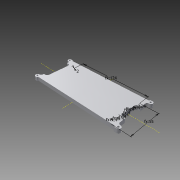
# Autodesk Inventor part: Heatsink
Saved by Autodesk Inventor 2016 (Build 200138000, 138)
## iProperties
Created: 2015-06-09
Part Number: Heatsink
Material: Aluminum 6061
Document SubType Name: Modeling
Designer: Yann
Density: 2.7 g/cm^3
Appearance: Aluminum - Flat
Mass: 133.784 g
Surface Area: 224.248 cm^2
Volume: 49.5496 cm^3
Author: Yann
Autodesk Inventor part; units mm, degrees
ref_plane "YZ Plane" through (0, 0, 0) normal (1, 0, 0) x (0, 1, 0)
ref_plane "XZ Plane" through (0, 0, 0) normal (0, 1, 0) x (-1, 0, 0)
ref_plane "XY Plane" through (0, 0, 0) normal (0, 0, 1) x (1, 0, 0)
sketch "Sketch1" plane through (0, 0, 0) normal (0, 0, 1) x (1, 0, 0)
  line L0 (0, 160210.1999) -> (0, -160210.1999) construction
  line L1 (-160320.9849, 0) -> (160320.9849, 0) construction
  line L2 (0, -32.5) -> (-72, -32.5)
  line L3 (-72, -32.5) -> (-72, -34.5)
  circle A0 centre (-75.5, -31) radius 1.5
  line L4 (-72, -34.5) -> (-75.5, -34.5)
  arc A1 (-75.7128, -27.5065) -> (-75.5, -34.5) centre (-75.5, -31) ccw
  line L5 (-72, -24.3936) -> (-72, 0) construction
  line L6 (-75.7128, -27.5065) -> (-72, -27.2803) construction
  line L7 (-72, -27.2803) -> (-72, -24.3936) construction
  spline S0 degree 2 poles (-75.7128, -27.5065) (-72, -27.2803) (-72, -24.3936) knots 1 1 1 2 2 2
  line L8 (0, -32.5) -> (72, -32.5)
  line L9 (72, -32.5) -> (72, -34.5)
  circle A2 centre (75.5, -31) radius 1.5
  line L10 (72, -34.5) -> (75.5, -34.5)
  arc A3 (75.5, -34.5) -> (75.7128, -27.5065) centre (75.5, -31) ccw
  line L11 (72, -24.3936) -> (72, 0) construction
  line L12 (75.7128, -27.5065) -> (72, -27.2803) construction
  line L13 (72, -27.2803) -> (72, -24.3936) construction
  spline S1 degree 2 poles (75.7128, -27.5065) (72, -27.2803) (72, -24.3936) knots 1 1 1 2 2 2
  line L14 (0, -160210.1999) -> (0, 160210.1999) construction
  line L15 (0, 32.5) -> (-72, 32.5)
  line L16 (-72, 32.5) -> (-72, 34.5)
  circle A4 centre (-75.5, 31) radius 1.5
  line L17 (-72, 34.5) -> (-75.5, 34.5)
  arc A5 (-75.5, 34.5) -> (-75.7128, 27.5065) centre (-75.5, 31) ccw
  line L18 (-72, 24.3936) -> (-72, 0) construction
  line L19 (-75.7128, 27.5065) -> (-72, 27.2803) construction
  line L20 (-72, 27.2803) -> (-72, 24.3936) construction
  spline S2 degree 2 poles (-75.7128, 27.5065) (-72, 27.2803) (-72, 24.3936) knots 1 1 1 2 2 2
  line L21 (0, 32.5) -> (72, 32.5)
  line L22 (72, 32.5) -> (72, 34.5)
  circle A6 centre (75.5, 31) radius 1.5
  line L23 (72, 34.5) -> (75.5, 34.5)
  arc A7 (75.7128, 27.5065) -> (75.5, 34.5) centre (75.5, 31) ccw
  line L24 (72, 24.3936) -> (72, 0) construction
  line L25 (75.7128, 27.5065) -> (72, 27.2803) construction
  spline S3 degree 2 poles (75.7128, 27.5065) (72, 27.2803) (72, 24.3936) knots 1 1 1 2 2 2
  line L26 (72, 27.2803) -> (72, 24.3936) construction
  line L27 (-72, -24.3936) -> (-72, -22)
  line L28 (-72, -22) -> (-69, -22)
  line L29 (-65, -18) -> (-65, 0)
  line L30 (-72, 24.3936) -> (-72, 22)
  line L31 (-72, 22) -> (-69, 22)
  line L32 (-65, 18) -> (-65, 0)
  line L33 (72, -24.3936) -> (72, -15)
  line L34 (72, -15) -> (69, -15)
  line L35 (65, -11) -> (65, 0)
  line L36 (72, 24.3936) -> (72, 15)
  line L37 (72, 15) -> (69, 15)
  line L38 (65, 11) -> (65, 0)
  arc A8 (-69, -22) -> (-65, -18) centre (-69, -18) ccw
  arc A9 (-65, 18) -> (-69, 22) centre (-69, 18) ccw
  arc A10 (69, 15) -> (65, 11) centre (69, 11) ccw
  arc A11 (65, -11) -> (69, -15) centre (69, -11) ccw
  point P0 (0, 0)
  point P1 (-65, -22)
  point P2 (-65, 22)
  point P3 (65, -15)
  point P4 (65, 15)
  dimension "d0" = 2
  dimension "d1" = 3
  dimension "d3" = 72
  dimension "d4" = 32.5
  dimension "d5" = 3.5
  dimension "d6" = 3.5
  dimension "d9" = 7
  dimension "d10" = 22
  dimension "d11" = 7
  dimension "d12" = 15
  dimension "d13" = 4
  constraints: 58 end point, 33 symmetric about line, 16 point on circle, 15 point on line, 12 centre point, 9 tangent, 4 coincident, 4 horizontal, 3 equal radius, 3 perpendicular, 2 vertical, 1 collinear, 19 other
  measures "d0" distance of L2.end L3.end
  measures "d1" diameter of A0
  measures "d3" distance of L2.start L2.end
  measures "d4" distance between parallel lines of L1 L2
  measures "d5" distance from line of A1.centre L3
  measures "d6" distance from line of L4 A0.centre
  measures "d9" distance of L27.end point (-65, -22)
  measures "d10" distance of point (-65, -22) L29.end
  measures "d11" distance of L33.end point (65, -15)
  measures "d12" distance of point (65, -15) L35.end
  measures "d13" radius of A8
extrude "Extrusion1" add sketch "Sketch1" against normal blind 7
sketch "Sketch2" plane through (0, 0, -7) normal (0, 0, -1) x (-1, 0, 0)
  line L0 (-110.6, 0) -> (110.6, 0) construction
  line L1 (0, -48.3) -> (0, 48.3) construction
  line L2 (-62, -27.5) -> (62, -27.5) construction
  line L3 (62, -27.5) -> (62, 27.5) construction
  line L4 (62, 27.5) -> (-62, 27.5) construction
  line L5 (-62, 27.5) -> (-62, -27.5) construction
  line L6 (62, -27.5) -> (-62, 27.5) construction
  line L7 (-62, -23.1242) -> (52.1345, 27.5) construction
  line L8 (-61.5945, -24.0383) -> (52.54, 26.5859)
  line L9 (51.7291, 28.4141) -> (-62.4055, -22.2101)
  arc A0 (-62.4055, -22.2101) -> (-61.5945, -24.0383) centre (-62, -23.1242) ccw
  arc A1 (52.54, 26.5859) -> (51.7291, 28.4141) centre (52.1345, 27.5) ccw
  line L10 (-62, -18.7484) -> (42.269, 27.5) construction
  line L11 (-61.5945, -19.6625) -> (42.6745, 26.5859)
  line L12 (41.8636, 28.4141) -> (-62.4055, -17.8343)
  arc A2 (-62.4055, -17.8343) -> (-61.5945, -19.6625) centre (-62, -18.7484) ccw
  arc A3 (42.6745, 26.5859) -> (41.8636, 28.4141) centre (42.269, 27.5) ccw
  line L13 (-62, -14.3726) -> (32.4036, 27.5) construction
  line L14 (-61.5945, -15.2867) -> (32.809, 26.5859)
  line L15 (31.9981, 28.4141) -> (-62.4055, -13.4584)
  arc A4 (-62.4055, -13.4584) -> (-61.5945, -15.2867) centre (-62, -14.3726) ccw
  arc A5 (32.809, 26.5859) -> (31.9981, 28.4141) centre (32.4036, 27.5) ccw
  line L16 (-62, -9.9967) -> (22.5381, 27.5) construction
  line L17 (-61.5945, -10.9109) -> (22.9436, 26.5859)
  line L18 (22.1326, 28.4141) -> (-62.4055, -9.0826)
  arc A6 (-62.4055, -9.0826) -> (-61.5945, -10.9109) centre (-62, -9.9967) ccw
  arc A7 (22.9436, 26.5859) -> (22.1326, 28.4141) centre (22.5381, 27.5) ccw
  line L19 (-62, -27.5) -> (62, 27.5) construction
  line L20 (-61.5945, -28.4141) -> (62.4055, 26.5859)
  line L21 (61.5945, 28.4141) -> (-62.4055, -26.5859)
  arc A8 (-62.4055, -26.5859) -> (-61.5945, -28.4141) centre (-62, -27.5) ccw
  arc A9 (62.4055, 26.5859) -> (61.5945, 28.4141) centre (62, 27.5) ccw
  line L22 (0, 0) -> (-4.9327, 2.1879) construction
  line L23 (-4.9327, 2.1879) -> (-9.8655, 4.3758) construction
  line L24 (-9.8655, 4.3758) -> (-14.7982, 6.5637) construction
  line L25 (-14.7982, 6.5637) -> (-19.731, 8.7516) construction
  line L26 (-62, -5.6209) -> (12.6726, 27.5) construction
  line L27 (-61.5945, -6.535) -> (13.0781, 26.5859)
  line L28 (12.2672, 28.4141) -> (-62.4055, -4.7068)
  arc A10 (-62.4055, -4.7068) -> (-61.5945, -6.535) centre (-62, -5.6209) ccw
  arc A11 (13.0781, 26.5859) -> (12.2672, 28.4141) centre (12.6726, 27.5) ccw
  line L29 (-62, -1.2451) -> (2.8071, 27.5) construction
  line L30 (-61.5945, -2.1592) -> (3.2126, 26.5859)
  line L31 (2.4017, 28.4141) -> (-62.4055, -0.331)
  arc A12 (-62.4055, -0.331) -> (-61.5945, -2.1592) centre (-62, -1.2451) ccw
  arc A13 (3.2126, 26.5859) -> (2.4017, 28.4141) centre (2.8071, 27.5) ccw
  line L32 (-62, 3.1307) -> (-7.0583, 27.5) construction
  line L33 (-61.5945, 2.2166) -> (-6.6529, 26.5859)
  line L34 (-7.4638, 28.4141) -> (-62.4055, 4.0448)
  arc A14 (-62.4055, 4.0448) -> (-61.5945, 2.2166) centre (-62, 3.1307) ccw
  arc A15 (-6.6529, 26.5859) -> (-7.4638, 28.4141) centre (-7.0583, 27.5) ccw
  line L35 (-62, 7.5065) -> (-16.9238, 27.5) construction
  line L36 (-61.5945, 6.5924) -> (-16.5183, 26.5859)
  line L37 (-17.3293, 28.4141) -> (-62.4055, 8.4206)
  arc A16 (-62.4055, 8.4206) -> (-61.5945, 6.5924) centre (-62, 7.5065) ccw
  arc A17 (-16.5183, 26.5859) -> (-17.3293, 28.4141) centre (-16.9238, 27.5) ccw
  line L38 (-62, 11.8823) -> (-26.7893, 27.5) construction
  line L39 (-61.5945, 10.9682) -> (-26.3838, 26.5859)
  line L40 (-27.1947, 28.4141) -> (-62.4055, 12.7965)
  arc A18 (-62.4055, 12.7965) -> (-61.5945, 10.9682) centre (-62, 11.8823) ccw
  arc A19 (-26.3838, 26.5859) -> (-27.1947, 28.4141) centre (-26.7893, 27.5) ccw
  line L41 (-62, 16.2582) -> (-36.6548, 27.5) construction
  line L42 (-61.5945, 15.344) -> (-36.2493, 26.5859)
  line L43 (-37.0602, 28.4141) -> (-62.4055, 17.1723)
  arc A20 (-62.4055, 17.1723) -> (-61.5945, 15.344) centre (-62, 16.2582) ccw
  arc A21 (-36.2493, 26.5859) -> (-37.0602, 28.4141) centre (-36.6548, 27.5) ccw
  line L44 (-62, 20.634) -> (-46.5202, 27.5) construction
  line L45 (-61.5945, 19.7199) -> (-46.1148, 26.5859)
  line L46 (-46.9257, 28.4141) -> (-62.4055, 21.5481)
  arc A22 (-62.4055, 21.5481) -> (-61.5945, 19.7199) centre (-62, 20.634) ccw
  arc A23 (-46.1148, 26.5859) -> (-46.9257, 28.4141) centre (-46.5202, 27.5) ccw
  line L47 (-62, 25.0098) -> (-56.3857, 27.5) construction
  line L48 (-61.5945, 24.0957) -> (-55.9802, 26.5859)
  line L49 (-56.7912, 28.4141) -> (-62.4055, 25.9239)
  arc A24 (-62.4055, 25.9239) -> (-61.5945, 24.0957) centre (-62, 25.0098) ccw
  arc A25 (-55.9802, 26.5859) -> (-56.7912, 28.4141) centre (-56.3857, 27.5) ccw
  point P0 (0, 0)
  point P1 (0, 0)
  point P2 (-24.6637, 10.9395)
  point P3 (-29.5964, 13.1274)
  point P4 (-34.5292, 15.3154)
  point P5 (-39.4619, 17.5033)
  point P6 (-44.3946, 19.6912)
  point P7 (-49.3274, 21.8791)
  point P8 (-54.2601, 24.067)
  point P9 (-59.1929, 26.2549)
  dimension "d15" = 124
  dimension "d16" = 55
  dimension "d17" = 2
  dimension "d18" = 4
  dimension "d19" = 4
  dimension "d20" = 4
  dimension "d21" = 4
  dimension "d22" = 4
  dimension "d23" = 4
  dimension "d25" = 4
  dimension "d26" = 4
  dimension "d27" = 4
  dimension "d28" = 4
  dimension "d29" = 4
  dimension "d30" = 4
  constraints: 118 end point, 52 point on circle, 52 tangent, 26 centre point, 25 parallel, 14 midpoint, 12 equal radius, 4 collinear, 2 coincident, 2 horizontal, 1 perpendicular, 1 vertical, 30 other
  measures "d15" distance of L3.end L6.end
  measures "d16" distance of L2.start L6.end
  measures "d17" diameter of A9
  measures "d18" distance between parallel lines of L7 L19
  measures "d19" distance between parallel lines of L10 L7
  measures "d20" distance between parallel lines of L13 L10
  measures "d21" distance between parallel lines of L16 L13
  measures "d22" distance between parallel lines of L26 L16
  measures "d23" distance between parallel lines of L29 L26
  measures "d25" distance between parallel lines of L32 L29
  measures "d26" distance between parallel lines of L35 L32
  measures "d27" distance between parallel lines of L38 L35
  measures "d28" distance between parallel lines of L41 L38
  measures "d29" distance between parallel lines of L44 L41
  measures "d30" distance between parallel lines of L44 L47
equation "\"d0\" = Cover_Thickness"
equation "\"d3\" = 0.5 * PowerPCB_Length + Interface_Thickness"
equation "\"d4\" = 0.5 * Heatsink_Width"
equation "\"d6\" = d5"
equation "\"d9\" = Interface_Thickness"
equation "\"d11\" = d9"
equation "\"d7\" = Heatsink_Thickness"
equation "\"d18\" = 2 * d17"
equation "\"d19\" = d18"
equation "\"d20\" = d18"
equation "\"d21\" = d18"
equation "\"d22\" = d18"
equation "\"d23\" = d18"
equation "\"d25\" = d18"
equation "\"d26\" = d18"
equation "\"d27\" = d18"
equation "\"d28\" = d18"
equation "\"d29\" = d18"
equation "\"d30\" = d18"
equation "\"Heatsink_Thickness\" = 7"
equation "\"Cover_Thickness\" = 2"
equation "\"Heatsink_Width\" = 65"
equation "\"Interface_Thickness\" = 7"
equation "\"PowerPCB_Minus_Height\" = 1.2"
equation "\"PowerPCB_Thickness\" = 3"
equation "\"PowerPCB_Plus_Height\" = 8"
equation "\"LogicPCB_Width\" = 55"
equation "\"LogicPCB_Thickness\" = 2"
equation "\"LogicPCB_Plus_Height\" = 8"
equation "\"HostPCB_Thickness\" = 1.2"
equation "\"HostPCB_Plus_Height\" = 8"
equation "\"PowerPCB_Length\" = 130"
body "Solid1"
